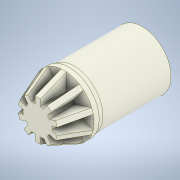
# Autodesk Inventor part: driver gear adapter
Saved by Autodesk Inventor 2022.6 (Build 266554000, 554)
## iProperties
Created: 2024-05-31
Part Number: driver gear adapter
Material: Generic
Document SubType Name: Modeling
Designer: david
Density: 1 g/cm^3
Appearance: Smooth - Ivory
Description: Custom printed Differential Gear
Mass: 1.2619 g
Surface Area: 12.5345 cm^2
Volume: 1.2619 cm^3
Author: david
Autodesk Inventor part; units mm, degrees
ref_plane "YZ Plane" through (0, 0, 0) normal (1, 0, 0) x (0, 1, 0)
ref_plane "XZ Plane" through (0, 0, 0) normal (0, 1, 0) x (-1, 0, 0)
ref_plane "XY Plane" through (0, 0, 0) normal (0, 0, 1) x (1, 0, 0)
sketch "Sketch1" plane through (0, 0, 0) normal (0, 0, 1) x (1, 0, 0)
  circle A0 centre (0, 0) radius 5.5
  dimension "d1" = 11
  constraints: 1 centre point, 1 coincident
  measures "d1" diameter of A0
extrude "Adapter" add sketch "Sketch1" along normal blind 1 and the other way blind 13
sketch "Sketch6" plane through (0, 0, -13) normal (0, 0, -1) x (-1, 0, 0)
  circle A0 centre (0, 0) radius 2.35
  line L0 (1.75, -1.5684) -> (-1.75, -1.5684)
  dimension "d35" = 4.7
  dimension "d92" = 3.5
  constraints: 2 end point, 2 point on circle, 1 centre point, 1 coincident, 1 horizontal
  measures "d35" diameter of A0
  measures "d92" distance of L0.start L0.end
extrude "Motor Shaft Profile" cut sketch "Sketch6" against normal blind 12 contours A0 L0 picked at (0.0927, -0.2678)
chamfer "Chamfer1" distance 0.5 angle 45 2 edges at (0, 2.35, -13) (0, -1.5684, -13)
thicken "Thicken5" [suppressed]
thicken "Thicken6" [suppressed]
sketch "Sketch9" plane through (-1.75, -1.5684, -1) normal (0, 1, 0) x (1, 0, 0)
  line L0 (0, 0) -> (3.5, 0) projected
  line L1 (1.75, 0) -> (1.75, 12) construction
  line L2 (7.25, 12) -> (-3.75, 12) projected
  point P0 (1.75, -1)
  point P1 (1.75, 6)
  constraints: 3 midpoint, 2 end point
hole "Hole6" at (0, -1.5684, -7) direction (0, -1, 0) diameter 2.85 end through all thread size "M3.5x0.6" class "6H" standard "ISO Metric profile"
sketch "Sketch10" plane through (0, 0, 1) normal (0, 0, 1) x (1, 0, 0)
  circle A0 centre (0, 0) radius 5.75
  dimension "d74" = 11.5
  constraints: 1 centre point, 1 coincident
  measures "d74" diameter of A0
extrude "Extrusion5" add sketch "Sketch10" along normal blind 1
sketch "Sketch11" plane through (0, 0, 0) normal (1, 0, 0) x (0, 1, 0)
  line L0 (5.75, 2) -> (-5.75, 2) projected
  line L1 (-5.75, 1) -> (-5.75, 2) projected
  line L2 (5.75, 1) -> (5.75, 2) projected
  line L3 (0, -16) -> (0, 5) projected
  line L4 (-5.75, 2) -> (-3.75, 7)
  line L5 (-3.75, 7) -> (0, 7)
  line L6 (5.75, 1) -> (-5.75, 1) projected
  line L7 (0, 7) -> (0, 2)
  point P0 (0, 0)
  dimension "d77" = 7.5
  dimension "d78" = 6
  constraints: 6 end point, 2 point on line, 1 midpoint, 1 perpendicular
  measures "d77" diameter of L4.end L3
  measures "d78" distance between parallel lines of L5 L6
extrude "Extrusion6" add sketch "Sketch11" along normal mid plane 1 contours L0 L4 L5 L7 L3
sketch "Sketch12" plane through (0, -5.75, 2) normal (0, 0, -1) x (-1, 0, 0)
  line L0 (0, 0) -> (0.5, 0) projected
  circle A0 centre (0, 5.75) radius 5.75 projected
  line L1 (0.5, 0.0218) -> (0.5, 0) projected
  line L2 (-0.5, 0) -> (0, 0) projected
  line L3 (-0.5, 0) -> (-0.5, 0.0218) projected
extrude "Extrusion7" cut sketch "Sketch12" against normal through all contours A0 L1 L0 | L2 L3 A0
pattern_circular "Circular Pattern1" count 10 over 360 about axis through (0, 0, -10) along (0, 0, 1) of "Extrusion6"
sketch "Sketch13" plane through (-0.5, -3.75, 7) normal (0, 0, 1) x (1, 0, 0)
  line L0 (1.9434, 6.25) -> (3.3868, 3.75)
  line L1 (3.3868, 3.75) -> (1.9434, 1.25)
  line L2 (1.9434, 1.25) -> (-0.9434, 1.25)
  line L3 (-0.9434, 1.25) -> (-2.3868, 3.75)
  line L4 (-2.3868, 3.75) -> (-0.9434, 6.25)
  line L5 (-0.9434, 6.25) -> (1.9434, 6.25)
  point P0 (0.5, 3.75)
  point P1 (0.5, 3.75)
  dimension "d86" = 5
  constraints: 12 end point, 1 coincident, 1 horizontal, 13 other
  measures "d86" distance between parallel lines of L2 L5
extrude "Extrusion8" add sketch "Sketch13" against normal up to surface (5 mm away)
fillet "Fillet1" radius 2 1 edges at (-5.5, 0, 1)
body "Solid1"
